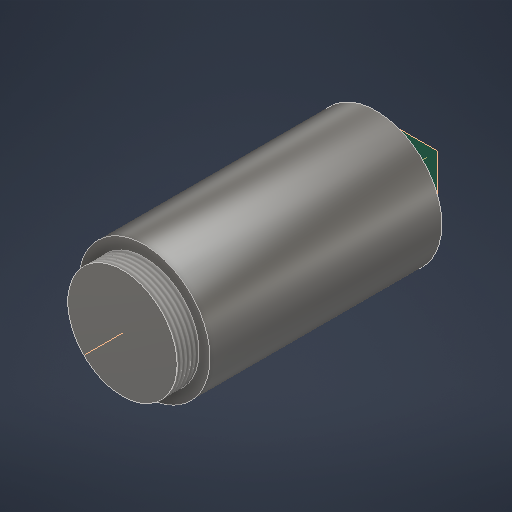
# Autodesk Inventor part: Nikon-Objektive-MUC11900_Mockup
Saved by Autodesk Inventor 2026 (Build 300175050, 175E)
## iProperties
Created: 2018-11-06
Part Number: Nikon-Objektive-MUC11900_Mockup
Material: Stainless Steel
Document SubType Name: Modeling
Designer: rainer
Density: 8 g/cm^3
Appearance: Semi-Polished
Mass: 334.106 g
Surface Area: 69.7874 cm^2
Volume: 41.7632 cm^3
Author: rainer
Autodesk Inventor part; units mm, degrees
ref_plane "YZ Plane" through (0, 0, 0) normal (1, 0, 0) x (0, 1, 0)
ref_plane "XZ Plane" through (0, 0, 0) normal (0, 1, 0) x (-1, 0, 0)
ref_plane "XY Plane" through (0, 0, 0) normal (0, 0, 1) x (1, 0, 0)
sketch "Sketch1" plane through (0, 0, 0) normal (0, 0, 1) x (1, 0, 0)
  circle A0 centre (0, 0) radius 15
  dimension "d0" = 30
  constraints: 1 centre point, 1 coincident
  measures "d0" diameter of A0
extrude "Extrusion1" add sketch "Sketch1" along normal blind 53
sketch "Sketch2" plane through (0, 0, 53) normal (0, 0, 1) x (1, 0, 0)
  circle A0 centre (0, 0) radius 12.5
  dimension "d3" = 25
  constraints: 1 centre point, 1 coincident
  measures "d3" diameter of A0
extrude "Extrusion2" add sketch "Sketch2" along normal blind 5
thread "Thread1" size "M25x1" class "6g" standard "ANSI Metric M Profile" length 25.006
sketch "Sketch3" plane through (0, 0, 0) normal (0, 0, -1) x (-1, 0, 0)
  circle A0 centre (0, 0) radius 6.5
  dimension "d8" = 13
  constraints: 1 centre point, 1 coincident
  measures "d8" diameter of A0
extrude "Extrusion3" add sketch "Sketch3" along normal blind 4.9
sketch "Sketch4" plane through (0, 0, 0) normal (0, 0, -1) x (-1, 0, 0)
  circle A0 centre (0, 0) radius 13.5
  dimension "d11" = 27
  constraints: 1 centre point, 1 coincident
  measures "d11" diameter of A0
extrude "Extrusion4" add sketch "Sketch4" along normal blind 2.5
sketch "Sketch5" plane through (0, 0, -2.5) normal (0, 0, -1) x (-1, 0, 0)
  circle A0 centre (0, 0) radius 10.15
  dimension "d14" = 20.3
  constraints: 1 centre point, 1 coincident
  measures "d14" diameter of A0
extrude "Extrusion5" add sketch "Sketch5" along normal blind 2.3
chamfer "Chamfer1" distance 1.5 angle 65 1 edges at (13.5, 0, -2.5) measured on face at (-13.3252, -2.1656, -1.6667)
chamfer "Chamfer2" distance 1.6 angle 65 1 edges at (10.15, 0, -4.8) measured on face at (-10.1171, -0.8167, -4.0333)
ref_plane "Work Plane1" through (0, 0, -6.9) normal (0, 0, -1) x (-1, 0, 0)
sketch "Sketch6" plane through (0, 0, 58) normal (0, 0, 1) x (1, 0, 0)
  circle A0 centre (0, 0) radius 10
  dimension "d24" = 20
  constraints: 1 centre point, 1 coincident
  measures "d24" diameter of A0
extrude "Extrusion6" cut sketch "Sketch6" against normal blind 58
sketch "Sketch7" plane through (0, 0, 0) normal (0, 0, 1) x (1, 0, 0)
  circle A0 centre (0, 0) radius 8
  dimension "d27" = 16
  constraints: 1 centre point, 1 coincident
  measures "d27" diameter of A0
extrude "Extrusion7" cut sketch "Sketch7" against normal blind 2
thicken "Thicken1" operation add thickness 58 both sides no extend neighbours no toward (0, 0, 1) faces at (9.159, -1.4359, 0)
thicken "Thicken2" operation add thickness 60 both sides no extend neighbours no toward (0, 0, 1) faces at (0.9456, 2.4934, -2)
body "Solid1"
